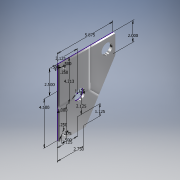
# Autodesk Inventor part: 15102898-16-P-0310
Saved by Autodesk Inventor 2017 (Build 210142000, 142)
## iProperties
Created: 2016-10-02
Part Number: 15102898-16-P-0310
Material: Aluminum 6061
Document SubType Name: Sheet Metal
Designer: gus
Density: 2.7 g/cm^3
Sheet Metal Rule: Default
Appearance: Aluminum - Flat
Mass: 362.619 g
Surface Area: 469.484 cm^2
Volume: 134.303 cm^3
Author: gus
Autodesk Inventor part; units mm, degrees
ref_plane "YZ Plane" through (0, 0, 0) normal (1, 0, 0) x (0, 1, 0)
ref_plane "XZ Plane" through (0, 0, 0) normal (0, 1, 0) x (-1, 0, 0)
ref_plane "XY Plane" through (0, 0, 0) normal (0, 0, 1) x (1, 0, 0)
sketch "Sketch1" plane through (0, 0, 0) normal (1, 0, 0) x (0, 1, 0)
  line L0 (0, 0) -> (63.5, 0)
  line L1 (63.5, 0) -> (63.5, -149.225)
  line L2 (63.5, -149.225) -> (12.7, -149.225)
  circle A0 centre (-31.75, -53.975) radius 14.2875
  line L3 (63.5, -25.4) -> (-43.502, -25.4) construction
  circle A1 centre (50.8, -12.7) radius 3.175
  circle A2 centre (-104.775, -12.7) radius 3.175
  line L4 (12.7, -149.225) -> (-114.3, -69.85)
  line L5 (-114.3, -69.85) -> (-114.3, 0)
  line L6 (-114.3, 0) -> (0, 0)
  circle A3 centre (-85.725, -53.975) radius 14.2875
  line L7 (-53.2384, 0) -> (-95.25, 0)
  circle A4 centre (-79.375, -12.7) radius 3.175
  circle A5 centre (25.4, -38.1) radius 3.175
  circle A6 centre (50.8, -63.5) radius 3.175
  circle A7 centre (22.225, -88.9) radius 3.175
  dimension "d1" = 28.575
  dimension "d2" = 63.5
  dimension "d6" = 25.4
  dimension "d7" = 6.35
  dimension "d8" = 6.35
  dimension "d9" = 12.7
  dimension "d10" = 12.7
  dimension "d12" = 12.7
  dimension "d17" = 50.8
  dimension "d18" = 114.3
  dimension "d19" = 9.525
  dimension "d20" = 53.975
  dimension "d21" = 28.575
  dimension "d24" = 53.975
  dimension "d25" = 69.85
  dimension "d26" = 53.975
  dimension "d27" = 149.225
  dimension "d28" = 107.002
  dimension "d45" = 6.35
  dimension "d46" = 12.7
  dimension "d47" = 25.4
  dimension "d48" = 6.35
  dimension "d49" = 38.1
  dimension "d50" = 38.1
  dimension "d53" = 6.35
  dimension "d54" = 6.35
  dimension "d55" = 41.275
  dimension "d56" = 88.9
  dimension "d57" = 12.7
  dimension "d58" = 63.5
  constraints: 16 end point, 8 centre point, 2 horizontal, 2 perpendicular, 2 point on line, 1 collinear, 1 equal radius, 1 parallel
  measures "d1" diameter of A0
  measures "d2" distance of L0.start L0.end
  measures "d6" distance between parallel lines of L0 L3
  measures "d7" diameter of A1
  measures "d8" diameter of A2
  measures "d9" distance from line of L3 A2.centre
  measures "d10" distance from line of L3 A1.centre
  measures "d12" distance from line of L1 A1.centre
  measures "d17" distance of L1.end L2.end
  measures "d18" distance from line of L0.start L5
  measures "d19" distance from line of L5 A2.centre
  measures "d20" distance from line of L6 A3.centre
  measures "d21" distance from line of L5 A3.centre
  measures "d24" distance from line of L0 A0.centre
  measures "d25" distance of L4.end L5.end
  measures "d26" distance of A3.centre A0.centre
  measures "d27" distance of L0.end L1.end
  measures "d28" distance of L3.start L3.end
  measures "d45" diameter of A4
  measures "d46" distance from line of L7 A4.centre
  measures "d47" distance of A2.centre A4.centre
  measures "d48" diameter of A5
  measures "d49" distance from line of L0 A5.centre
  measures "d50" distance from line of L1 A5.centre
  measures "d53" diameter of A7
  measures "d54" diameter of A6
  measures "d55" distance from line of L1 A7.centre
  measures "d56" distance from line of L0 A7.centre
  measures "d57" distance from line of L1 A6.centre
  measures "d58" distance from line of L0 A6.centre
extrude "Extrusion1" add sketch "Sketch1" along normal blind 6.35 contours L0 L1 L2 L4 L5 L6 | A3 | A4 | A5 | A6 | A7
sketch "Sketch2" plane through (0, 0, 0) normal (-1, 0, 0) x (0, 0, 1)
  circle A0 centre (-127, 38.1) radius 14.2875
  line L0 (-149.225, 63.5) -> (-149.225, 12.7) projected
  line L1 (0, 63.5) -> (-149.225, 63.5) projected
  point P0 (0, 0)
  dimension "d40" = 28.575
  dimension "d41" = 22.225
  dimension "d42" = 25.4
  constraints: 1 centre point
  measures "d40" diameter of A0
  measures "d41" distance from line of L0 A0.centre
  measures "d42" distance from line of L1 A0.centre
extrude "Extrusion3" cut sketch "Sketch2" against normal blind 25.4
extrude "Extrusion4" cut sketch "Sketch1" along normal blind 25.4 contours A4 | A5 | A6 | A7
equation "\"BendRadius\" = Thickness"
equation "\"BendReliefWidth\" = Thickness"
equation "\"BendReliefDepth\" = 0.5 * Thickness"
equation "\"CornerReliefSize\" = 4 * Thickness"
equation "\"MinimumRemnant\" = 2 * Thickness"
equation "\"TransitionRadius\" = BendRadius"
equation "\"JacobiRadiusSize\" = Thickness"
equation "\"GapSize\" = Thickness"
equation "\"Thickness\" = 3.048"
body "Solid1"
